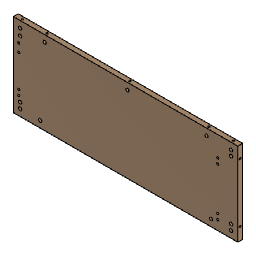
Y mounting board (Autodesk Fusion 360 design; units mm, degrees)
Autodesk Fusion 360 part; units mm, degrees
sketch "Front" plane through (0, 0, 0) normal (0, 1, 0) x (1, 0, 0)
  line L0 (420, -155.75) -> (-420, -155.75)
  line L1 (-420, -155.75) -> (-420, 155.75)
  line L2 (-420, 155.75) -> (420, 155.75)
  line L3 (420, 155.75) -> (420, -155.75)
  line L4 (420, -155.75) -> (-420, 155.75) construction
  line L5 (-420, -155.75) -> (420, 155.75) construction
  line L6 (-395, -155.75) -> (-395, 155.75) construction
  line L7 (-400, -100) -> (-400, 110) construction
  line L8 (-420, -130.75) -> (420, -130.75) construction
  circle A0 centre (-395, -130.75) radius 6
  circle A1 centre (-303, -130.75) radius 6
  circle A2 centre (-395, -105.75) radius 6
  circle A3 centre (-400, -80) radius 4
  circle A4 centre (-400, -50) radius 4
  circle A5 centre (-400, 90) radius 4
  circle A6 centre (-400, 70) radius 4
  line L9 (-420, 130.75) -> (420, 130.75) construction
  circle A7 centre (-395, 130.75) radius 6
  circle A8 centre (-320, 130.75) radius 6
  circle A9 centre (-395, 109.25) radius 6
  line L10 (395, -155.75) -> (395, 155.75) construction
  circle A10 centre (395, -130.75) radius 6
  circle A11 centre (395, 130.75) radius 6
  circle A12 centre (395, -110.75) radius 6
  circle A13 centre (303, -130.75) radius 6
  circle A14 centre (395, 109.25) radius 6
  circle A15 centre (320, 130.75) radius 6
  line L11 (345, -120) -> (345, 120) construction
  circle A16 centre (345, -80) radius 4
  circle A17 centre (345, -60) radius 4
  circle A18 centre (345, 100) radius 4
  circle A19 centre (345, 120) radius 4
  circle A20 centre (7, -130.75) radius 6
  dimension "d1" = 840
  dimension "d2" = 311.5
  dimension "d3" = 25
  dimension "d4" = 5
  dimension "d5" = 25
  dimension "d6" = 12
  dimension "d7" = 12
  dimension "d8" = 12
  dimension "d9" = 92
  dimension "d10" = 25
  dimension "d11" = 8
  dimension "d12" = 8
  dimension "d13" = 30
  dimension "d14" = 25.75
  dimension "d15" = 8
  dimension "d16" = 8
  dimension "d17" = 25
  dimension "d18" = 12
  dimension "d19" = 12
  dimension "d20" = 75
  dimension "d21" = 20
  dimension "d22" = 120
  dimension "d23" = 12
  dimension "d24" = 215
  dimension "d25" = 25
  dimension "d26" = 12
  dimension "d27" = 12
  dimension "d28" = 12
  dimension "d29" = 12
  dimension "d30" = 12
  dimension "d31" = 12
  dimension "d32" = 50
  dimension "d33" = 8
  dimension "d34" = 8
  dimension "d35" = 8
  dimension "d36" = 8
  dimension "d37" = 20
  dimension "d38" = 20
  dimension "d39" = 160
  dimension "d40" = 75.75
  dimension "d41" = 75.75
  dimension "d42" = 92
  dimension "d43" = 20
  dimension "d44" = 220
  dimension "d45" = 75
  dimension "d46" = 12
  dimension "d47" = 310
  dimension "d48" = 296
  constraint perpendicular L0 L1
  constraint parallel L0 L2
  constraint parallel L1 L3
  constraint horizontal L0
  constraint coincident L4 origin
  constraint coincident L5 origin
  constraint coincident L0 L6.start
  constraint coincident L2 L6.end
  constraint perpendicular L2 L6
  constraint parallel L6 L7
  constraint coincident L1 L8.start
  constraint coincident L3 L8.end
  constraint perpendicular L3 L8
  constraint coincident L6 A0.centre
  constraint coincident L8 A0.centre
  constraint coincident L8 A1.centre
  constraint coincident L6 A2.centre
  constraint coincident L7 A3.centre
  constraint coincident L7 A4.centre
  constraint coincident L7 A5.centre
  constraint coincident L7 A6.centre
  constraint perpendicular L6 L9
  constraint coincident L6 A7.centre
  constraint coincident L9 A7.centre
  constraint coincident L9 A8.centre
  constraint coincident L6 A9.centre
  constraint coincident L0 L10.start
  constraint coincident L2 L10.end
  constraint perpendicular L2 L10
  constraint coincident L8 A10.centre
  constraint coincident L10 A10.centre
  constraint coincident L10 A11.centre
  constraint coincident L9 A11.centre
  constraint coincident L10 A12.centre
  constraint coincident L8 A13.centre
  constraint coincident L10 A14.centre
  constraint coincident L9 A15.centre
  constraint vertical L11
  constraint coincident L11 A16.centre
  constraint coincident L11 A17.centre
  constraint coincident L11 A18.centre
  constraint coincident L11 A19.centre
  constraint coincident L8 A20.centre
  measures "d1" distance of L1.end L2.end
  measures "d2" distance of L0.end L1.end
  measures "d3" distance of L1 L6
  measures "d4" distance of L6 L7
  measures "d5" distance of L0 L8
  measures "d6" diameter of A0
  measures "d7" diameter of A1
  measures "d8" diameter of A2
  measures "d9" distance of A0.centre A1.centre
  measures "d10" distance of A0.centre A2.centre
  measures "d11" diameter of A3
  measures "d12" diameter of A4
  measures "d13" distance of A3.centre A4.centre
  measures "d14" vertical distance of A2.centre A3.centre
  measures "d15" diameter of A5
  measures "d16" diameter of A6
  measures "d17" distance of L2 L9
  measures "d18" diameter of A7
  measures "d19" diameter of A8
  measures "d20" distance of A7.centre A8.centre
  measures "d21" distance of A5.centre A6.centre
  measures "d22" distance of A4.centre A6.centre
  measures "d23" diameter of A9
  measures "d24" distance of A2.centre A9.centre
  measures "d25" distance of L3 L10
  measures "d26" diameter of A10
  measures "d27" diameter of A11
  measures "d28" diameter of A12
  measures "d29" diameter of A13
  measures "d30" diameter of A14
  measures "d31" diameter of A15
  measures "d32" distance of L10 L11
  measures "d33" diameter of A16
  measures "d34" diameter of A17
  measures "d35" diameter of A18
  measures "d36" diameter of A19
  measures "d37" distance of A16.centre A17.centre
  measures "d38" distance of A18.centre L11.end
  measures "d39" distance of A17.centre A18.centre
  measures "d40" distance of L0 A3.centre
  measures "d41" distance of L0 A16.centre
  measures "d42" distance of A10.centre A13.centre
  measures "d43" distance of A10.centre A12.centre
  measures "d44" distance of A12.centre A14.centre
  measures "d45" distance of A11.centre A15.centre
  measures "d46" diameter of A20
  measures "d47" distance of A1.centre A20.centre
  measures "d48" distance of A13.centre A20.centre
extrude "Extrude1" add sketch "Front" against normal blind 18
sketch "Top" plane through (0, 0, 155.75) normal (0, 0, 1) x (-1, 0, 0)
  line L0 (-420, 0) -> (420, 0)
  line L1 (420, 0) -> (420, 18)
  line L2 (420, 18) -> (-420, 18)
  line L3 (-420, 18) -> (-420, 0)
  line L4 (420, 9) -> (-420, 9) construction
  line L5 (395, 17) -> (395, 1) construction
  line L6 (303, 17) -> (303, 1) construction
  line L7 (-7, 17) -> (-7, 1) construction
  line L8 (-303, 17) -> (-303, 1) construction
  line L9 (-395, 17) -> (-395, 1) construction
  circle A0 centre (395, 9) radius 3.5
  circle A1 centre (303, 9) radius 3.5
  circle A2 centre (-7, 9) radius 3.5
  circle A3 centre (-303, 9) radius 3.5
  circle A4 centre (-395, 9) radius 3.5
  dimension "d51" = 92
  dimension "d52" = 296
  dimension "d53" = 310
  dimension "d54" = 92
  dimension "d55" = 25
  dimension "d56" = 7
  dimension "d57" = 7
  dimension "d58" = 7
  dimension "d59" = 7
  dimension "d60" = 7
  dimension "d61" = 25
  constraint midpoint L1 L4.start
  constraint midpoint L3 L4.end
  constraint perpendicular L4 L5
  constraint perpendicular L4 L6
  constraint perpendicular L4 L7
  constraint perpendicular L4 L8
  constraint perpendicular L4 L9
  constraint midpoint L5 A0.centre
  constraint midpoint L6 A1.centre
  constraint midpoint L7 A2.centre
  constraint midpoint L8 A3.centre
  constraint midpoint L9 A4.centre
  measures "d51" distance of L8 L9
  measures "d52" distance of L7 L8
  measures "d53" distance of L6 L7
  measures "d54" distance of L5 L6
  measures "d55" distance of L1 L5
  measures "d56" diameter of A0
  measures "d57" diameter of A1
  measures "d58" diameter of A2
  measures "d59" diameter of A3
  measures "d60" diameter of A4
  measures "d61" distance of L3 A4.centre
extrude "Extrude2" cut sketch "Top" against normal blind 35 contours A0 | A1 | A2 | A3 | A4
sketch "Right" plane through (420, 0, 0) normal (1, 0, 0) x (0, 1, 0)
  line L0 (0, -155.75) -> (0, 155.75)
  line L1 (0, 155.75) -> (-18, 155.75)
  line L2 (-18, 155.75) -> (-18, -155.75)
  line L3 (-18, -155.75) -> (0, -155.75)
  line L4 (-9, 155.75) -> (-9, -155.75) construction
  line L5 (0, 110.75) -> (-18, 110.75) construction
  line L6 (0, -109.25) -> (-18, -109.25) construction
  circle A0 centre (-9, 110.75) radius 3.5
  circle A1 centre (-9, -109.25) radius 3.5
  dimension "d64" = 220
  dimension "d65" = 45
  dimension "d66" = 7
  dimension "d67" = 7
  constraint midpoint L1 L4.start
  constraint midpoint L3 L4.end
  constraint coincident L0 L5.start
  constraint coincident L2 L5.end
  constraint perpendicular L2 L5
  constraint coincident L0 L6.start
  constraint coincident L2 L6.end
  constraint perpendicular L2 L6
  constraint midpoint L5 A0.centre
  constraint midpoint L6 A1.centre
  measures "d64" distance of L5 L6
  measures "d65" distance of L1 L5
  measures "d66" diameter of A0
  measures "d67" diameter of A1
extrude "Extrude3" cut sketch "Right" against normal blind 35 contours A0 | A1
sketch "Left" plane through (-420, 0, 0) normal (-1, 0, 0) x (0, -1, 0)
  line L0 (0, 155.75) -> (0, -155.75)
  line L1 (0, -155.75) -> (18, -155.75)
  line L2 (18, -155.75) -> (18, 155.75)
  line L3 (18, 155.75) -> (0, 155.75)
  line L4 (9, 155.75) -> (9, -155.75) construction
  line L5 (0, 105.75) -> (18, 105.75) construction
  line L6 (0, -109.25) -> (18, -109.25) construction
  circle A0 centre (9, 105.75) radius 3.5
  circle A1 centre (9, -109.25) radius 3.5
  dimension "d70" = 215
  dimension "d71" = 50
  dimension "d72" = 7
  dimension "d73" = 7
  constraint midpoint L3 L4.start
  constraint midpoint L1 L4.end
  constraint coincident L2 L5.end
  constraint perpendicular L2 L5
  constraint coincident L0 L6.start
  constraint coincident L2 L6.end
  constraint perpendicular L4 L6
  constraint midpoint L5 A0.centre
  constraint midpoint L6 A1.centre
  measures "d70" distance of L5 L6
  measures "d71" distance of L3 L5
  measures "d72" diameter of A0
  measures "d73" diameter of A1
extrude "Extrude4" cut sketch "Left" against normal blind 35 contours A0 | A1
sketch "Bottom" plane through (0, 0, -155.75) normal (0, 0, -1) x (1, 0, 0)
  line L0 (-420, 0) -> (420, 0)
  line L1 (420, 0) -> (420, 18)
  line L2 (420, 18) -> (-420, 18)
  line L3 (-420, 18) -> (-420, 0)
  line L4 (-420, 9) -> (420, 9) construction
  line L5 (395, 18) -> (395, 0) construction
  line L6 (320, 18) -> (320, 0) construction
  line L7 (-320, 0) -> (-320, 18) construction
  line L8 (-395, 0) -> (-395, 18) construction
  circle A0 centre (395, 9) radius 3.5
  circle A1 centre (320, 9) radius 3.5
  circle A2 centre (-320, 9) radius 3.5
  circle A3 centre (-395, 9) radius 3.5
  dimension "d76" = 75
  dimension "d77" = 25
  dimension "d78" = 25
  dimension "d79" = 75
  dimension "d80" = 7
  dimension "d81" = 7
  dimension "d82" = 7
  dimension "d83" = 7
  constraint midpoint L3 L4.start
  constraint midpoint L1 L4.end
  constraint coincident L2 L5.start
  constraint coincident L0 L5.end
  constraint perpendicular L0 L5
  constraint coincident L2 L6.start
  constraint coincident L0 L6.end
  constraint perpendicular L0 L6
  constraint coincident L0 L7.start
  constraint coincident L2 L7.end
  constraint perpendicular L2 L7
  constraint coincident L0 L8.start
  constraint coincident L2 L8.end
  constraint perpendicular L4 L8
  constraint midpoint L5 A0.centre
  constraint midpoint L6 A1.centre
  constraint midpoint L7 A2.centre
  constraint midpoint L8 A3.centre
  measures "d76" distance of L7 L8
  measures "d77" distance of L3 L8
  measures "d78" distance of L1 L5
  measures "d79" distance of L5 L6
  measures "d80" diameter of A0
  measures "d81" diameter of A1
  measures "d82" diameter of A2
  measures "d83" diameter of A3
extrude "Extrude5" cut sketch "Bottom" against normal blind 35 contours A2 | A3
extrude "Extrude6" cut sketch "Bottom" against normal blind 35 contours A0 | A1
named bodies: "Board"
